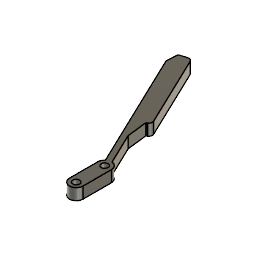
Finger (Autodesk Fusion 360 design; units mm, degrees)
part number: 2026-03-10-23-15-20-442
Autodesk Fusion 360 part; units mm, degrees
sketch "Sketch1" plane through (0, 0, 0) normal (0, 0, 1) x (1, 0, 0)
  line L0 (59.3493, -22.9672) -> (59.3493, -47.9176)
  arc A0 (59.3493, -47.9176) -> (71.3493, -47.9176) centre (65.3493, -47.9176) ccw
  line L1 (71.3493, -47.9176) -> (71.3493, -22.9672)
  arc A1 (71.3493, -22.9672) -> (59.3493, -22.9672) centre (65.3493, -22.9672) ccw
  line L2 (65.3493, -22.9672) -> (65.3493, -47.9176) construction
  line L3 (61.4359, -18.4191) -> (12.6813, 83.5221)
  line L4 (12.6813, 83.5221) -> (13.3354, 93.4004)
  line L5 (13.3354, 93.4004) -> (20.0498, 95.3795)
  line L6 (23.6044, 93.7962) -> (53.1349, 32.0506)
  arc A2 (23.6044, 93.7962) -> (20.0498, 95.3795) centre (20.898, 92.5019) ccw
  line L7 (65.8452, -17.0002) -> (52.9015, 10.0639)
  line L8 (51.7229, 28.0498) -> (50.8208, 27.6184)
  line L9 (50.8208, 27.6184) -> (52.9015, 10.0639)
  arc A3 (51.7229, 28.0498) -> (53.1349, 32.0506) centre (50.4285, 30.7562) ccw
  point P0 (22.5016, 96.1021)
  point P1 (54.4293, 29.3442)
  dimension "d1" = 12
  dimension "d2" = 113
  dimension "d3" = 154.44
  dimension "d4" = 74
  dimension "d5" = 9.9
  dimension "d7" = 3
  dimension "d8" = 7
  dimension "d9" = 30
  dimension "d10" = 4.59
  dimension "d11" = 3
  dimension "d12" = 1
  constraint tangent L0 A0
  constraint tangent A0 L1
  constraint parallel L0 L1
  constraint tangent L1 A1
  constraint tangent L0 A1
  constraint vertical L2
  constraint parallel L3 L6
  constraint coincident P0 L5
  constraint coincident P0 L6
  constraint tangent L5 A2
  constraint tangent L6 A2
  constraint parallel L3 L7
  constraint perpendicular L6 L8
  constraint coincident A1 L3.start
  constraint coincident P1 L8
  constraint coincident P1 L6
  constraint tangent L8 A3
  constraint tangent L6 A3
  measures "d1" diameter of A0
  measures "d2" distance of L3.start L3.end
  measures "d3" angle of L0 L3
  measures "d4" distance of P0 P1
  measures "d5" distance of L3.end L4.end
  measures "d7" radius of A2
  measures "d8" distance of L4.end L5.end
  measures "d9" distance of L7.start L7.end
  measures "d10" distance of L3 L7
  measures "d11" radius of A3
  measures "d12" distance of L8.end L8.start
extrude "Extrude1" add sketch "Sketch1" along normal blind 10
sketch "Sketch2" plane through (0, 0, 10) normal (0, 0, 1) x (-1, 0, 0)
  line L0 (-50.8208, -27.6184) -> (-51.7229, -28.0498)
  arc A0 (-51.7229, -28.0498) -> (-53.1349, -32.0506) centre (-50.4285, -30.7562) ccw
  line L1 (-53.1349, -32.0506) -> (-23.6044, -93.7962)
  arc A1 (-23.6044, -93.7962) -> (-20.0498, -95.3795) centre (-20.898, -92.5019) ccw
  line L2 (-20.0498, -95.3795) -> (-13.3354, -93.4004)
  line L3 (-13.3354, -93.4004) -> (-12.6813, -83.5221)
  line L4 (-12.6813, -83.5221) -> (-61.4359, 18.4191)
  arc A2 (-61.4359, 18.4191) -> (-59.3493, 22.9672) centre (-65.3493, 22.9672) ccw
  line L5 (-59.3493, 22.9672) -> (-59.3493, 47.9176)
  arc A3 (-59.3493, 47.9176) -> (-71.3493, 47.9176) centre (-65.3493, 47.9176) ccw
  line L6 (-71.3493, 47.9176) -> (-71.3493, 22.9672)
  arc A4 (-71.3493, 22.9672) -> (-65.839, 16.9872) centre (-65.3493, 22.9672) ccw
  line L7 (-65.839, 16.9872) -> (-52.9015, -10.0639)
  line L8 (-52.9015, -10.0639) -> (-50.8208, -27.6184)
  circle A5 centre (-65.3493, 22.9672) radius 3
  circle A6 centre (-65.3493, 47.9176) radius 3
  dimension "d15" = 6
  dimension "d16" = 6
  constraint concentric A2 A5
  constraint concentric A3 A6
  measures "d15" diameter of A5
  measures "d16" diameter of A6
extrude "Extrude2" cut sketch "Sketch2" against normal blind 30 contours A5 | A6
